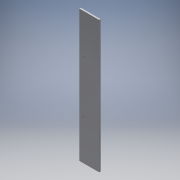
# Autodesk Inventor part: model 2 comp 2 floor part 1
Saved by Autodesk Inventor 2017 (Build 210142000, 142)
## iProperties
Created: 2017-06-12
Part Number: model 2 comp 2 floor part 1
Material: Generic
Document SubType Name: Modeling
Designer: cas7
Density: 1 g/cm^3
Appearance: Default
Author: cas7
Autodesk Inventor part; units mm, degrees
ref_plane "YZ Plane" through (0, 0, 0) normal (1, 0, 0) x (0, 1, 0)
ref_plane "XZ Plane" through (0, 0, 0) normal (0, 1, 0) x (-1, 0, 0)
ref_plane "XY Plane" through (0, 0, 0) normal (0, 0, 1) x (1, 0, 0)
sketch "Sketch2" plane through (0, 0, 0) normal (0, 0, 1) x (1, 0, 0)
  line L0 (0, 0) -> (209.55, 0)
  line L1 (209.55, 0) -> (209.55, 1397)
  line L2 (209.55, 1397) -> (0, 1397)
  line L3 (0, 1397) -> (0, 0)
  dimension "d4" = 209.55
  dimension "d5" = 1397
  constraints: 8 end point, 2 parallel, 1 horizontal, 1 perpendicular
  measures "d4" distance of L2.end L1.end
  measures "d5" distance of L1.end L0.end
extrude "Extrusion2" add sketch "Sketch2" along normal blind 15.875
sketch "Sketch4" plane through (0, 0, 15.875) normal (0, 0, 1) x (1, 0, 0)
  line L0 (0, 1397) -> (0, 0) projected
  line L1 (0, 971.55) -> (44.45, 971.55)
  line L2 (44.45, 971.55) -> (44.45, 425.45)
  dimension "d18" = 44.45
  constraints: 4 end point, 2 coincident, 1 horizontal, 1 perpendicular, 1 point on line
  measures "d18" distance of L1.start L1.end
hole "Hole2" at (44.45, 971.55, 15.875) at (44.45, 425.45, 15.875) direction (0, 0, -1) diameter 10.5918 end through all thread size "1/2-13 UNC" class "2B" standard "ANSI Unified Screw Threads"
body "Solid2"
